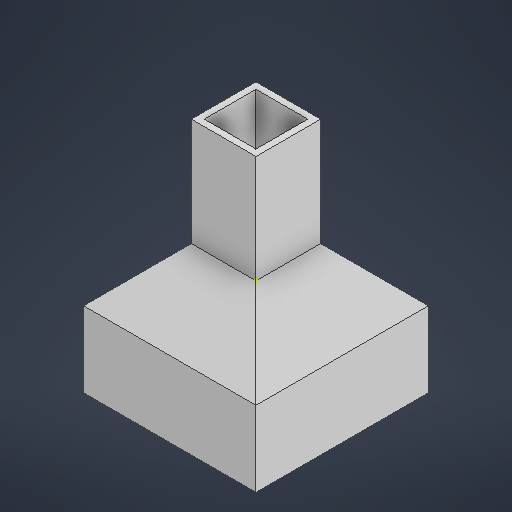
# Autodesk Inventor part: tolva
Saved by Autodesk Inventor 2026.1 (Build 301233020, 233B)
## iProperties
Created: 2025-12-03
Part Number: tolva
Material: Genérico
Document SubType Name: Modeling
Designer: benja
Density: 1 g/cm^3
Appearance: Valor por defecto
Author: benja
Autodesk Inventor part; units mm, degrees
ref_plane "YZ Plane" through (0, 0, 0) normal (1, 0, 0) x (0, 1, 0)
ref_plane "XZ Plane" through (0, 0, 0) normal (0, 1, 0) x (-1, 0, 0)
ref_plane "XY Plane" through (0, 0, 0) normal (0, 0, 1) x (1, 0, 0)
sketch "Boceto1" plane through (0, 0, 0) normal (0, 1, 0) x (-1, 0, 0)
  line L0 (0, 0) -> (30, 0)
  line L1 (30, 0) -> (30, -30)
  line L2 (30, -30) -> (0, -30)
  line L3 (0, -30) -> (0, 0)
  dimension "d0" = 30
  dimension "d1" = 30
  constraints: 8 end point, 2 parallel, 1 horizontal, 1 perpendicular
  measures "d0" distance of L1.end L2.end
  measures "d1" distance of L0.end L1.end
extrude "Extrusión1" add sketch "Boceto1" along normal blind 50
sketch "Boceto2" plane through (0, 50, 0) normal (0, 1, 0) x (1, 0, 0)
  line L0 (-30, 0) -> (0, 0) projected
  line L1 (0, 0) -> (-3, 0)
  line L2 (-3, 0) -> (-6, 0)
  line L3 (-3, 0) -> (-3, 3)
  line L4 (-30, 30) -> (-30, 0) projected
  line L5 (-30, 30) -> (-27, 30)
  line L6 (0, 30) -> (-30, 30) projected
  line L7 (-27, 30) -> (-30, 30)
  line L8 (-27, 30) -> (-27, 27)
  line L9 (-3, 3) -> (-27, 3)
  line L10 (-27, 3) -> (-27, 27)
  line L11 (-27, 27) -> (-3, 27)
  line L12 (-3, 27) -> (-3, 3)
  dimension "d4" = 3
  dimension "d6" = 3
  dimension "d7" = 3
  dimension "d8" = 3
  dimension "d9" = 3
  constraints: 20 end point, 3 point on line, 2 parallel, 2 vertical, 1 collinear, 1 horizontal, 1 perpendicular
  measures "d4" distance of L0.end L1.end
  measures "d6" distance of L1.end L3.end
  measures "d7" distance of L4.start L5.end
  measures "d8" distance of L5.end L4.start
  measures "d9" distance of L5.end L8.end
extrude "Extrusión2" cut sketch "Boceto2" against normal blind 184.25 contours L9 L10 L11 L12
sketch "Boceto3" plane through (0, 0, 0) normal (1, 0, 0) x (0, 0, -1)
  point P0 (0, 0)
sketch "Boceto4" plane through (0, 0, 0) normal (0, -1, 0) x (1, 0, 0)
  line L0 (25, 25) -> (-55, 25)
  line L1 (-55, 25) -> (-55, -55)
  line L2 (-55, -55) -> (25, -55)
  line L3 (25, -55) -> (25, 25)
  line L4 (25, -55) -> (25, -15)
  line L5 (25, -15) -> (-15, -15)
  line L6 (0, 0) -> (0, -30) projected
  line L7 (0, 0) -> (0, -15)
  line L8 (0, -15) -> (-15, -15)
  dimension "d12" = 80
  dimension "d13" = 80
  dimension "d14" = 40
  dimension "d15" = 40
  dimension "d16" = 15
  dimension "d17" = 15
  constraints: 16 end point, 3 perpendicular, 2 midpoint, 2 parallel, 1 horizontal
  measures "d12" distance of L2.end L1.end
  measures "d13" distance of L1.end L0.end
  measures "d14" distance of L2.end L4.end
  measures "d15" distance of L4.end L5.end
  measures "d16" distance of L6.start L7.end
  measures "d17" distance of L7.end L8.end
extrude "Extrusión3" add sketch "Boceto4" along normal blind 60
chamfer "Chaflán1" distance 25 angle 45 1 edges at (-55, 0, -15)
chamfer "Chaflán2" distance 25 angle 45 1 edges at (-2.5003, 0, 25)
chamfer "Chaflán3" distance 25 angle 45 1 edges at (-2.5003, 0, -55)
chamfer "Chaflán4" distance 25 angle 45 1 edges at (25, 0, -15)
sketch "Boceto6" plane through (0, -60, 0) normal (0, -1, 0) x (1, 0, 0)
  line L0 (0, 0) -> (25, 25) projected
  line L1 (-55, -55) -> (-30, -30) projected
  line L2 (15.6406, 15.6406) -> (-47.7087, 15.6406)
  line L3 (-47.7087, 15.6406) -> (-47.7087, -47.7087)
  line L4 (-47.7087, -47.7087) -> (15.6406, -47.7087)
  line L5 (15.6406, -47.7087) -> (15.6406, 15.6406)
  constraints: 8 end point, 2 parallel, 2 point on line, 1 horizontal, 1 perpendicular
extrude "Extrusión5" cut sketch "Boceto6" against normal blind 40.25
sketch "Boceto7" plane through (0, 0, 0) normal (0, 1, 0) x (1, 0, 0)
  line L0 (-3, 27) -> (-27, 27) projected
  line L1 (-3, 3) -> (-3, 27) projected
  line L2 (-27, 27) -> (-3, 27)
  line L3 (-3, 27) -> (-3, 3)
  line L4 (-3, 3) -> (-27, 3)
  line L5 (-27, 3) -> (-27, 27)
  point P0 (0, 0)
  constraints: 8 end point, 2 parallel, 1 horizontal, 1 perpendicular
extrude "Extrusión6" cut sketch "Boceto7" against normal blind 184.25
chamfer "Chaflán5" distance 18 angle 45 4 edges at (-27, -19.75, -15) (-15, -19.75, -3) (-15, -19.75, -27) (-3, -19.75, -15)
